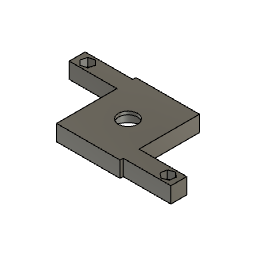
Right Rack n Rod Connector (Autodesk Fusion 360 design; units mm, degrees)
Autodesk Fusion 360 part; units mm, degrees
sketch "Top" plane through (0, 0, 0) normal (0, 0, 1) x (1, 0, 0)
  line L0 (0, 0) -> (40, 0)
  line L1 (40, 0) -> (40, 50)
  line L2 (40, 50) -> (0, 50)
  line L3 (0, 50) -> (0, 0)
  circle A0 centre (20, 25) radius 11.2
  circle A1 centre (20, 25) radius 6
  dimension "d6" = 40
  dimension "d7" = 50
  dimension "d11" = 22.4
  dimension "d12" = 25
  dimension "d13" = 20
  dimension "d27" = 12
  constraint horizontal L0
  constraint vertical L1
  constraint horizontal L2
  constraint vertical L3
  constraint coincident L0.start L3.end
  constraint concentric A0 A1
  measures "d6" distance of L0.start L0.end
  measures "d7" distance of L0.start L2.end
  measures "d11" diameter of A0
  measures "d12" distance of L2 A0.centre
  measures "d13" distance of L1 A0.centre
  measures "d27" diameter of A1
extrude "Extrude1" add sketch "Top" along normal blind 10 contours L0 L1 L2 L3 | A0 | A1
extrude "Extrude2" cut sketch "Top" along normal blind 8 contours A0 | A1
extrude "Extrude5" cut sketch "Top" along normal blind 110 contours A1
sketch "Sketch5" plane through (0, 0, 0) normal (-1, 0, 0) x (0, -1, 0)
  line L0 (-50, 0) -> (0, 0)
  line L1 (0, 0) -> (0, 10)
  line L2 (0, 10) -> (-50, 10)
  line L3 (-50, 10) -> (-50, 0)
  line L4 (-48, 10) -> (-38, 10)
  line L5 (-38, 10) -> (-38, 0)
  line L6 (-38, 0) -> (-48, 0)
  line L7 (-48, 0) -> (-48, 10)
  dimension "d50" = 10
  dimension "d51" = 10
  dimension "d52" = 2
  constraint horizontal L4
  constraint vertical L5
  constraint horizontal L6
  constraint vertical L7
  constraint coincident L2 L4.start
  measures "d50" distance of L4.start L4.end
  measures "d51" distance of L4.start L6.end
  measures "d52" distance of L3 L7
extrude "Extrude8" add sketch "Sketch5" along normal blind 30 contours L0 L2 L4 L5 L6 L7
sketch "Sketch8" plane through (40, 0, 0) normal (1, 0, 0) x (0, 1, 0)
  line L0 (0, 0) -> (50, 0)
  line L1 (50, 0) -> (50, 10)
  line L2 (50, 10) -> (0, 10)
  line L3 (0, 10) -> (0, 0)
  line L4 (2, 10) -> (12, 10)
  line L5 (12, 10) -> (12, 0)
  line L6 (12, 0) -> (2, 0)
  line L7 (2, 0) -> (2, 10)
  dimension "d72" = 10
  dimension "d73" = 10
  dimension "d74" = 2
  constraint horizontal L4
  constraint vertical L5
  constraint horizontal L6
  constraint vertical L7
  constraint coincident L2 L4.start
  measures "d72" distance of L4.start L6.end
  measures "d73" distance of L4.start L4.end
  measures "d74" distance of L3 L7
extrude "Extrude11" add sketch "Sketch8" along normal blind 30 contours L0 L2 L4 L5 L6 L7
sketch "Sketch10" plane through (0, 0, 10) normal (0, 0, 1) x (-1, 0, 0)
  circle A0 centre (-20, -25) radius 6
  line L0 (0, -50) -> (0, -48)
  line L1 (0, -48) -> (30, -48)
  line L2 (30, -48) -> (30, -38)
  line L3 (30, -38) -> (0, -38)
  line L4 (0, -38) -> (0, 0)
  line L5 (0, 0) -> (-40, 0)
  line L6 (-40, 0) -> (-40, -2)
  line L7 (-40, -2) -> (-70, -2)
  line L8 (-70, -2) -> (-70, -12)
  line L9 (-70, -12) -> (-40, -12)
  line L10 (-40, -12) -> (-40, -50)
  line L11 (-40, -50) -> (0, -50)
  line L12 (20.5049, -40.1716) -> (19.4696, -44.0353)
  line L13 (19.4696, -44.0353) -> (22.2981, -46.8637)
  line L14 (22.2981, -46.8637) -> (26.1618, -45.8284)
  line L15 (26.1618, -45.8284) -> (27.197, -41.9647)
  line L16 (27.197, -41.9647) -> (24.3686, -39.1363)
  line L17 (24.3686, -39.1363) -> (20.5049, -40.1716)
  line L18 (-67.0472, -8.4856) -> (-63.9038, -10.9591)
  line L19 (-63.9038, -10.9591) -> (-60.1898, -9.4736)
  line L20 (-60.1898, -9.4736) -> (-59.6194, -5.5144)
  line L21 (-59.6194, -5.5144) -> (-62.7629, -3.0409)
  line L22 (-62.7629, -3.0409) -> (-66.4768, -4.5264)
  line L23 (-66.4768, -4.5264) -> (-67.0472, -8.4856)
  point P0 (23.3333, -43)
  point P1 (-63.3333, -7)
  dimension "d93" = 4
  dimension "d94" = 5
  dimension "d95" = 6.6667
  dimension "d96" = 4
  dimension "d97" = 6.6667
  dimension "d98" = 5
  measures "d93" distance of L12.start P0
  measures "d94" distance of L3 P0
  measures "d95" distance of L2 P0
  measures "d96" distance of L18.start P1
  measures "d97" distance of L8 P1
  measures "d98" distance of L7 P1
extrude "Extrude13" cut sketch "Sketch10" against normal blind 5 contours L12 L13 L14 L15 L16 L17 | L18 L19 L20 L21 L22 L23
equation "length = 50 mm"
equation "width = 40 mm"
equation "thickness = 10 mm"
equation "extra = 100 mm"
equation "fit_gap = 0.2 mm"
equation "d6 = width"
equation "d7 = length"
equation "d8 = thickness"
equation "bearing_outer_radius = 11.1 mm"
equation "d11 = ( bearing_outer_radius * 2 ) + fit_gap"
equation "d12 = length / 2"
equation "d13 = width / 2"
equation "d14 = thickness - 2 mm"
equation "bearing_inner_radius = ( 8 mm + 4 mm ) / 2"
equation "d27 = bearing_inner_radius * 2"
equation "d28 = thickness + extra"
equation "rack_rock_bracket_length = 30 mm"
equation "rack_rock_bracket_width = 10 mm"
equation "rack_rock_bracket_big_distance = 2 mm"
equation "d50 = rack_rock_bracket_width"
equation "d51 = rack_rock_bracket_width"
equation "d52 = rack_rock_bracket_big_distance"
equation "d53 = rack_rock_bracket_length"
equation "d72 = rack_rock_bracket_width"
equation "d73 = rack_rock_bracket_width"
equation "d74 = rack_rock_bracket_big_distance"
equation "d75 = rack_rock_bracket_length"
equation "bearing_dowel_radius = 0.8 mm"
equation "bearing_dowel_length = 10 mm"
equation "bearing_dowel_big_distance = 2 mm + bearing_dowel_radius"
equation "bearing_dowel_small_distance = rack_rock_bracket_width / 2"
equation "polygon_dowel_hole_side_length = 4 mm"
equation "polygon_dowel_hole_height = 5 mm"
equation "polygon_dowel_small_distance = thickness / 2"
equation "polygon_dowel_big_distance = polygon_dowel_small_distance + ( polygon_dowel_small_distance / 3 )"
equation "d93 = polygon_dowel_hole_side_length"
equation "d94 = polygon_dowel_small_distance"
equation "d95 = polygon_dowel_big_distance"
equation "d96 = polygon_dowel_hole_side_length"
equation "d97 = polygon_dowel_big_distance"
equation "d98 = polygon_dowel_small_distance"
equation "d99 = -polygon_dowel_hole_height"
